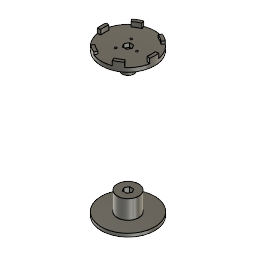
HexapodStand (Autodesk Fusion 360 design; units mm, degrees)
Autodesk Fusion 360 part; units mm, degrees
sketch "Tyc" plane through (0, 0, 0) normal (0, 0, 1) x (1, 0, 0)
  circle A0 centre (0, 0) radius 6
  line L0 (6, 0) -> (3, 5.1962)
  line L1 (3, 5.1962) -> (-3, 5.1962)
  line L2 (-3, 5.1962) -> (-6, 0)
  line L3 (-6, 0) -> (-3, -5.1962)
  line L4 (-3, -5.1962) -> (3, -5.1962)
  line L5 (3, -5.1962) -> (6, 0)
  dimension "d1" = 12
  constraint coincident A0.centre origin
  constraint coincident A0 L0.start
  constraint horizontal L1
  measures "d1" diameter of A0
extrude "Extrude1" add sketch "Tyc" along normal blind 214 contours L0 L1 L2 L3 L4 L5 makes body 1
copy_body "Body->Comp1" bodies 1 removing the originals makes body 2 in component "Tyc"
sketch "Podstava" plane through (0, 0, 0) normal (0, 0, -1) x (1, 0, 0)
  circle A0 centre (0, 0) radius 40
  circle A1 centre (0, 0) radius 16.05
  line L0 (6, 0) -> (3, 5.1962)
  line L1 (3, 5.1962) -> (-3, 5.1962)
  line L2 (-3, 5.1962) -> (-6, 0)
  line L3 (-6, 0) -> (-3, -5.1962)
  line L4 (-3, -5.1962) -> (3, -5.1962)
  line L5 (3, -5.1962) -> (6, 0)
  line L6 (6, 0) -> (3, 5.1962)
  line L7 (3, 5.1962) -> (-3, 5.1962)
  line L8 (-3, 5.1962) -> (-6, 0)
  line L9 (-6, 0) -> (-3, -5.1962)
  line L10 (-3, -5.1962) -> (3, -5.1962)
  line L11 (3, -5.1962) -> (6, 0)
  dimension "d6" = 80
  dimension "d8" = 32.1
  constraint coincident A0.centre A1.centre
  measures "d6" diameter of A0
  measures "d8" diameter of A1
extrude "Extrude2" add sketch "Podstava" against normal blind 5 separate body contours A0 makes body 3
copy_body "Body->Comp2" bodies 3 removing the originals makes body 4 in component "Podstava"
extrude "Extrude1'" add sketch "Podstava" against normal blind 33 contours A1 bodies 4 in component "Podstava"
sketch "Nasada" plane through (0, 0, 214) normal (0, 0, 1) x (-1, 0, 0)
  line L0 (-3, 5.1962) -> (-6, 0)
  line L1 (-6, 0) -> (-3, -5.1962)
  line L2 (-3, -5.1962) -> (3, -5.1962)
  line L3 (3, -5.1962) -> (6, 0)
  line L4 (6, 0) -> (3, 5.1962)
  line L5 (3, 5.1962) -> (-3, 5.1962)
  circle A0 centre (0, 0) radius 18
  circle A1 centre (-13.5, 0) radius 1.5
  circle A2 centre (-13.5, 0) radius 3
  line L6 (0, 0) -> (-13.5, 0)
  circle A3 centre (6.75, -11.6913) radius 1.5
  circle A4 centre (6.75, -11.6913) radius 3
  circle A5 centre (6.75, 11.6913) radius 1.5
  circle A6 centre (6.75, 11.6913) radius 3
  circle A7 centre (0, 0) radius 9
  dimension "d16" = 36
  dimension "d19" = 3
  dimension "d20" = 6
  dimension "d22" = 13.5
  dimension "d24" = 360
  dimension "d29" = 18
  constraint coincident A0.centre L6.start
  constraint concentric A1 A2
  constraint horizontal L6
  constraint coincident A1.centre A2.centre
  measures "d16" diameter of A0
  measures "d19" diameter of A1
  measures "d20" diameter of A2
  measures "d22" distance of A0.centre A1.centre
  measures "d29" diameter of A7
extrude "Extrude3" add sketch "Nasada" against normal blind 6 separate body contours A0 | A7 makes body 5
extrude "Extrude4" add sketch "Nasada" against normal blind 3 contours A2 | A4 | A6 bodies 5
extrude "Extrude5" add sketch "Nasada" against normal blind 26 contours A7 bodies 5
copy_body "Body->Comp3" bodies 5 removing the originals makes body 6 in component "Nasada"
sketch "Drzak" plane through (0, 0, 214) normal (0, 0, 1) x (-1, 0, 0)
  line L0 (-3, 5.1962) -> (-6, 0)
  line L1 (-6, 0) -> (-3, -5.1962)
  line L2 (-3, -5.1962) -> (3, -5.1962)
  line L3 (3, -5.1962) -> (6, 0)
  line L4 (6, 0) -> (3, 5.1962)
  line L5 (3, 5.1962) -> (-3, 5.1962)
  circle A0 centre (0, 0) radius 40
  circle A1 centre (0, 0) radius 35
  line L6 (0, 0) -> (-39.3923, 6.9459)
  line L7 (0, 0) -> (-39.3923, -6.9459)
  line L8 (0, 0) -> (-40, 0)
  line L9 (0, 0) -> (-13.6808, -37.5877)
  line L10 (0, 0) -> (-25.7115, -30.6418)
  line L11 (0, 0) -> (25.7115, -30.6418)
  line L12 (0, 0) -> (13.6808, -37.5877)
  line L13 (0, 0) -> (39.3923, 6.9459)
  line L14 (0, 0) -> (39.3923, -6.9459)
  line L15 (0, 0) -> (13.6808, 37.5877)
  line L16 (0, 0) -> (25.7115, 30.6418)
  line L17 (0, 0) -> (-25.7115, 30.6418)
  line L18 (0, 0) -> (-13.6808, 37.5877)
  circle A2 centre (6.75, 11.6913) radius 1.5
  circle A3 centre (-13.5, 0) radius 1.5
  circle A4 centre (6.75, -11.6913) radius 1.5
  dimension "d32" = 80
  dimension "d33" = 70
  dimension "d34" = 10
  dimension "d35" = 10
  dimension "d37" = 360
  constraint coincident A0.centre A1.centre
  constraint concentric A0 A1
  constraint coincident A0 L6.end
  constraint coincident A0 L7.end
  constraint coincident A0 L8.end
  constraint horizontal L8
  measures "d32" diameter of A0
  measures "d33" diameter of A1
  measures "d34" angle of L6 L8
  measures "d35" angle of L7 L8
extrude "Extrude1''" add sketch "Drzak" along normal blind 6 separate body contours L0 L5 A1 L17 L18 | L0 A1 L6 L17 | L5 A1 L15 L18 | L0 A1 L6 L8 A3 | A0 A1 L17 L18 | A0 A1 L6 L17 | L4 L5 A1 L15 L16 | A0 A1 L15 L18 | L1 A1 L7 L8 A3 | A0 A1 L6 L8 | L1 A1 L7 L10 | L1 L2 A1 L9 L10 | L2 A1 L9 L12 | L2 L3 A1 L11 L12 | L3 A1 L11 L14 | L3 L4 A1 L13 L14 | L4 A1 L13 L16 | A0 A1 L15 L16 | A0 A1 L7 L8 | A0 A1 L7 L10 | A0 A1 L9 L10 | A0 A1 L9 L12 | A0 A1 L11 L12 | A0 A1 L11 L14 | A0 A1 L13 L14 | A0 A1 L13 L16 makes body 7 in component "Drzak"
extrude "Extrude2'" add sketch "Drzak" along normal blind 13 contours A0 A1 L17 L18 | A0 A1 L6 L8 | A0 A1 L7 L8 | A0 A1 L11 L12 | A0 A1 L13 L14 bodies 7 in component "Drzak"
extrude "Extrude3'" add sketch "Drzak" along normal blind 10 contours A0 A1 L15 L16 | A0 A1 L9 L10 bodies 7 in component "Drzak"
move_face "OffsetFaces1" offset -0.179 6 faces at (-1, -5.1962, 216) (-5, -1.7321, 216) (5, 1.7321, 216) (4, -3.4641, 216) (-4, 3.4641, 216) (1, 5.1962, 216) on bodies 7 in component "Drzak"
move_face "OffsetFaces1'" offset -0.179 6 faces at (-5, 1.7321, 11) (-1, 5.1962, 22) (5, -1.7321, 22) (4, 3.4641, 11) (-4, -3.4641, 11) (1, -5.1962, 22) on bodies 4 in component "Podstava"
move_face "OffsetFaces1''" offset -0.179 6 faces at (1, -5.1962, 196.6667) (-5, -1.7321, 205.3333) (4, -3.4641, 205.3333) (5, 1.7321, 205.3333) (1, 5.1962, 205.3333) (-4, 3.4641, 205.3333) on bodies 6 in component "Nasada"
move_face "OffsetFaces2" offset -0.15 19 faces at (-22.6243, 32.987, 220.3333) (-13.1108, -36.0216, 221.3333) (-20.3522, -28.4743, 221.3333) (-23.5689, -28.0883, 221.3333) (14.4834, -31.8627, 222.3333) (13.1108, -36.0216, 224.6667) (24.6402, -29.365, 224.6667) (-36.1096, 6.3671, 222.3333) (-34.678, 4.7366, 222.3333) (-12.5407, 34.4554, 222.3333) (36.1096, 6.3671, 222.3333) (14.4834, 31.8627, 222.6667) (-20.3522, 28.4743, 222.3333) (-23.5689, 28.0883, 222.3333) (-36.1096, -6.3671, 222.3333) (36.1096, -6.3671, 222.3333) (34.9934, 0.6787, 222.3333) (23.5689, 28.0883, 221.3333) (13.1108, 36.0216, 221.3333) on bodies 7 in component "Drzak"
component "Tyc" placed x (1, 0, 0) y (0, 1, 0) z (0, 0, 1) at (0, 0, 0)
component "Drzak" placed x (1, 0, 0) y (0, 1, 0) z (0, 0, 1) at (0, 0, 0)
component "Podstava" placed x (1, 0, 0) y (0, 1, 0) z (0, 0, 1) at (0, 0, 0)
component "Nasada" placed x (1, 0, 0) y (0, 1, 0) z (0, 0, 1) at (0, 0, 0)
equation "d1 = PrumerTyce"
equation "PrumerTyce = 12 mm"
equation "DelkaTyce = 214 mm"
equation "d4 = DelkaTyce"
equation "d6 = PrumerPodstavy"
equation "PrumerPodstavy = 80 mm"
equation "d8 = PrumerOtvoruCinky"
equation "PrumerOtvoruCinky = 32.1 mm"
equation "VyskaPodstavy = 5 mm"
equation "VyskaOtvoruCinky = 28 mm"
equation "d12 = -VyskaPodstavy"
equation "d14 = -VyskaPodstavy - VyskaOtvoruCinky"
equation "d16 = PrumerNasady"
equation "PrumerNasady = 36 mm"
equation "Tloustka = 6 mm"
equation "d30 = -6 mm - 20 mm"
equation "d40 = 6 mm + 7 mm"
equation "d42 = 6 mm + 4 mm"
named bodies: "Tyc"
